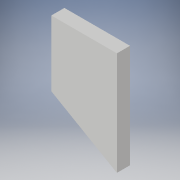
# Autodesk Inventor part: top right door
Saved by Autodesk Inventor 2017 (Build 210142000, 142)
## iProperties
Created: 2018-03-10
Part Number: top right door
Material: Generic
Document SubType Name: Modeling
Designer: Braxton
Density: 1 g/cm^3
Appearance: Default
Author: Braxton
Autodesk Inventor part; units mm, degrees
ref_plane "YZ Plane" through (0, 0, 0) normal (1, 0, 0) x (0, 1, 0)
ref_plane "XZ Plane" through (0, 0, 0) normal (0, 1, 0) x (-1, 0, 0)
ref_plane "XY Plane" through (0, 0, 0) normal (0, 0, 1) x (1, 0, 0)
sketch "Sketch1" plane through (0, 0, 0) normal (0, 0, 1) x (1, 0, 0)
  line L0 (1270, 1270) -> (1270, 2540)
  line L1 (1270, 1270) -> (2540, 536.7652)
  line L2 (2540, 536.7652) -> (2540, 2540)
  line L3 (2540, 2540) -> (1270, 2540)
  dimension "d448" = 2003.2348
  constraints: 8 end point
  measures "d448" distance of L1.end L2.end
extrude "door" add sketch "Sketch1" along normal mid plane 254
sketch "Sketch3" plane through (0, 0, 0) normal (0, 0, 1) x (1, 0, 0)
  line L0 (1295.4, 2436.0832) -> (1270, 2407.6852)
  line L1 (1295.4, 2461.4832) -> (1295.4, 2436.0832)
  line L2 (1270, 2448.7832) -> (1295.4, 2448.7832) construction
  line L3 (1270, 2489.8813) -> (1270, 2407.6852)
  line L4 (1270, 2489.8813) -> (1295.4, 2461.4832)
  line L5 (1295.4, 2271.691) -> (1270, 2243.2929)
  line L6 (1295.4, 2297.091) -> (1295.4, 2271.691)
  line L7 (1270, 2284.391) -> (1295.4, 2284.391) construction
  line L8 (1270, 2325.4891) -> (1270, 2243.2929)
  line L9 (1270, 2325.4891) -> (1295.4, 2297.091)
  line L10 (1244.6, 2353.8871) -> (1270, 2325.4891)
  line L11 (1270, 2366.5871) -> (1244.6, 2366.5871) construction
  line L12 (1244.6, 2379.2871) -> (1244.6, 2353.8871)
  line L13 (1244.6, 2379.2871) -> (1270, 2407.6852)
  line L14 (1270, 2407.6852) -> (1270, 2325.4891)
  line L15 (1295.4, 2107.2987) -> (1270, 2078.9007)
  line L16 (1295.4, 2132.6987) -> (1295.4, 2107.2987)
  line L17 (1270, 2119.9987) -> (1295.4, 2119.9987) construction
  line L18 (1270, 2161.0968) -> (1270, 2078.9007)
  line L19 (1270, 2161.0968) -> (1295.4, 2132.6987)
  line L20 (1244.6, 2189.4949) -> (1270, 2161.0968)
  line L21 (1270, 2202.1949) -> (1244.6, 2202.1949) construction
  line L22 (1244.6, 2214.8949) -> (1244.6, 2189.4949)
  line L23 (1244.6, 2214.8949) -> (1270, 2243.2929)
  line L24 (1270, 2243.2929) -> (1270, 2161.0968)
  line L25 (1295.4, 1942.9065) -> (1270, 1914.5084)
  line L26 (1295.4, 1968.3065) -> (1295.4, 1942.9065)
  line L27 (1270, 1955.6065) -> (1295.4, 1955.6065) construction
  line L28 (1270, 1996.7045) -> (1270, 1914.5084)
  line L29 (1270, 1996.7045) -> (1295.4, 1968.3065)
  line L30 (1244.6, 2025.1026) -> (1270, 1996.7045)
  line L31 (1270, 2037.8026) -> (1244.6, 2037.8026) construction
  line L32 (1244.6, 2050.5026) -> (1244.6, 2025.1026)
  line L33 (1244.6, 2050.5026) -> (1270, 2078.9007)
  line L34 (1270, 2078.9007) -> (1270, 1996.7045)
  line L35 (1295.4, 1778.5142) -> (1270, 1750.1162)
  line L36 (1295.4, 1803.9142) -> (1295.4, 1778.5142)
  line L37 (1270, 1791.2142) -> (1295.4, 1791.2142) construction
  line L38 (1270, 1832.3123) -> (1270, 1750.1162)
  line L39 (1270, 1832.3123) -> (1295.4, 1803.9142)
  line L40 (1244.6, 1860.7104) -> (1270, 1832.3123)
  line L41 (1270, 1873.4104) -> (1244.6, 1873.4104) construction
  line L42 (1244.6, 1886.1104) -> (1244.6, 1860.7104)
  line L43 (1244.6, 1886.1104) -> (1270, 1914.5084)
  line L44 (1270, 1914.5084) -> (1270, 1832.3123)
  line L45 (1295.4, 1614.122) -> (1270, 1585.7239)
  line L46 (1295.4, 1639.522) -> (1295.4, 1614.122)
  line L47 (1270, 1626.822) -> (1295.4, 1626.822) construction
  line L48 (1270, 1667.92) -> (1270, 1585.7239)
  line L49 (1270, 1667.92) -> (1295.4, 1639.522)
  line L50 (1244.6, 1696.3181) -> (1270, 1667.92)
  line L51 (1270, 1709.0181) -> (1244.6, 1709.0181) construction
  line L52 (1244.6, 1721.7181) -> (1244.6, 1696.3181)
  line L53 (1244.6, 1721.7181) -> (1270, 1750.1162)
  line L54 (1270, 1750.1162) -> (1270, 1667.92)
  line L55 (1295.4, 1449.7297) -> (1270, 1421.3317)
  line L56 (1295.4, 1475.1297) -> (1295.4, 1449.7297)
  line L57 (1270, 1462.4297) -> (1295.4, 1462.4297) construction
  line L58 (1270, 1503.5278) -> (1270, 1421.3317)
  line L59 (1270, 1503.5278) -> (1295.4, 1475.1297)
  line L60 (1244.6, 1531.9258) -> (1270, 1503.5278)
  line L61 (1270, 1544.6258) -> (1244.6, 1544.6258) construction
  line L62 (1244.6, 1557.3258) -> (1244.6, 1531.9258)
  line L63 (1244.6, 1557.3258) -> (1270, 1585.7239)
  line L64 (1270, 1585.7239) -> (1270, 1503.5278)
  line L65 (1244.6, 1392.9336) -> (1270, 1421.3317)
  line L66 (1270, 1380.2336) -> (1244.6, 1380.2336) construction
  line L67 (1244.6, 1392.9336) -> (1244.6, 1367.5336)
  line L68 (1270, 1421.3317) -> (1270, 1339.1355)
  line L69 (1244.6, 1367.5336) -> (1270, 1339.1355)
  line L70 (2540, 536.7652) -> (1270, 1270) projected
  line L71 (1531.5315, 1148.3341) -> (1543.4249, 1112.138)
  line L72 (1507.833, 1132.6871) -> (1520.533, 1154.6841) construction
  line L73 (1531.5315, 1148.3341) -> (1509.5344, 1161.0341)
  line L74 (1543.4249, 1112.138) -> (1472.241, 1153.2361)
  line L75 (1509.5344, 1161.0341) -> (1472.241, 1153.2361)
  line L76 (1472.241, 1153.2361) -> (1434.9475, 1145.4381)
  line L77 (1436.649, 1173.7851) -> (1423.949, 1151.7881) construction
  line L78 (1434.9475, 1145.4381) -> (1412.9505, 1158.1381)
  line L79 (1389.1636, 1230.5302) -> (1401.0571, 1194.3342)
  line L80 (1389.1636, 1230.5302) -> (1367.1666, 1243.2302)
  line L81 (1401.0571, 1194.3342) -> (1329.8731, 1235.4322)
  line L82 (1365.4651, 1214.8832) -> (1378.1651, 1236.8802) construction
  line L83 (1412.9505, 1158.1381) -> (1401.0571, 1194.3342)
  line L84 (1472.241, 1153.2361) -> (1401.0571, 1194.3342)
  line L85 (1367.1666, 1243.2302) -> (1329.8731, 1235.4322)
  line L86 (2267.1577, 664.9613) -> (2255.2643, 701.1574)
  line L87 (2289.1548, 652.2613) -> (2267.1577, 664.9613)
  line L88 (2290.8562, 680.6084) -> (2278.1562, 658.6113) construction
  line L89 (2326.4482, 660.0593) -> (2255.2643, 701.1574)
  line L90 (2326.4482, 660.0593) -> (2289.1548, 652.2613)
  line L91 (2243.3708, 737.3535) -> (2255.2643, 701.1574)
  line L92 (2219.6723, 721.7064) -> (2232.3723, 743.7035) construction
  line L93 (2243.3708, 737.3535) -> (2221.3738, 750.0535)
  line L94 (2255.2643, 701.1574) -> (2184.0803, 742.2555)
  line L95 (2221.3738, 750.0535) -> (2184.0803, 742.2555)
  line L96 (2184.0803, 742.2555) -> (2146.7869, 734.4575)
  line L97 (2148.4884, 762.8045) -> (2135.7884, 740.8075) construction
  line L98 (2146.7869, 734.4575) -> (2124.7898, 747.1575)
  line L99 (2124.7898, 747.1575) -> (2112.8964, 783.3535)
  line L100 (2184.0803, 742.2555) -> (2112.8964, 783.3535)
  line L101 (2101.003, 819.5496) -> (2112.8964, 783.3535)
  line L102 (2077.3044, 803.9026) -> (2090.0044, 825.8996) construction
  line L103 (2101.003, 819.5496) -> (2079.0059, 832.2496)
  line L104 (2112.8964, 783.3535) -> (2041.7125, 824.4516)
  line L105 (2041.7125, 824.4516) -> (2004.419, 816.6536)
  line L106 (2006.1205, 845.0006) -> (1993.4205, 823.0036) construction
  line L107 (2004.419, 816.6536) -> (1982.422, 829.3536)
  line L108 (1982.422, 829.3536) -> (1970.5285, 865.5497)
  line L109 (2041.7125, 824.4516) -> (1970.5285, 865.5497)
  line L110 (2079.0059, 832.2496) -> (2041.7125, 824.4516)
  line L111 (1958.6351, 901.7457) -> (1970.5285, 865.5497)
  line L112 (1934.9366, 886.0987) -> (1947.6366, 908.0957) construction
  line L113 (1958.6351, 901.7457) -> (1936.638, 914.4457)
  line L114 (1970.5285, 865.5497) -> (1899.3446, 906.6477)
  line L115 (1899.3446, 906.6477) -> (1862.0512, 898.8497)
  line L116 (1863.7526, 927.1968) -> (1851.0526, 905.1997) construction
  line L117 (1862.0512, 898.8497) -> (1840.0541, 911.5497)
  line L118 (1840.0541, 911.5497) -> (1828.1607, 947.7458)
  line L119 (1899.3446, 906.6477) -> (1828.1607, 947.7458)
  line L120 (1936.638, 914.4457) -> (1899.3446, 906.6477)
  line L121 (1816.2672, 983.9419) -> (1828.1607, 947.7458)
  line L122 (1792.5687, 968.2948) -> (1805.2687, 990.2919) construction
  line L123 (1816.2672, 983.9419) -> (1794.2702, 996.6419)
  line L124 (1828.1607, 947.7458) -> (1756.9767, 988.8439)
  line L125 (1794.2702, 996.6419) -> (1756.9767, 988.8439)
  line L126 (1756.9767, 988.8439) -> (1719.6833, 981.0458)
  line L127 (1721.3848, 1009.3929) -> (1708.6848, 987.3958) construction
  line L128 (1719.6833, 981.0458) -> (1697.6862, 993.7458)
  line L129 (1697.6862, 993.7458) -> (1685.7928, 1029.9419)
  line L130 (1756.9767, 988.8439) -> (1685.7928, 1029.9419)
  line L131 (1673.8994, 1066.138) -> (1685.7928, 1029.9419)
  line L132 (1650.2008, 1050.4909) -> (1662.9008, 1072.488) construction
  line L133 (1673.8994, 1066.138) -> (1651.9023, 1078.838)
  line L134 (1685.7928, 1029.9419) -> (1614.6089, 1071.04)
  line L135 (1651.9023, 1078.838) -> (1614.6089, 1071.04)
  line L136 (1579.0169, 1091.589) -> (1566.3169, 1069.592) construction
  line L137 (1577.3154, 1063.242) -> (1555.3184, 1075.942)
  line L138 (1555.3184, 1075.942) -> (1543.4249, 1112.138)
  line L139 (1614.6089, 1071.04) -> (1543.4249, 1112.138)
  line L140 (1614.6089, 1071.04) -> (1577.3154, 1063.242)
  line L141 (2409.5256, 582.7652) -> (2397.6321, 618.9613)
  line L142 (2431.5226, 570.0652) -> (2409.5256, 582.7652)
  line L143 (2433.2241, 598.4123) -> (2420.5241, 576.4152) construction
  line L144 (2468.8161, 577.8632) -> (2397.6321, 618.9613)
  line L145 (2468.8161, 577.8632) -> (2431.5226, 570.0652)
  line L146 (2385.7387, 655.1574) -> (2397.6321, 618.9613)
  line L147 (2362.0402, 639.5103) -> (2374.7402, 661.5074) construction
  line L148 (2363.7416, 667.8574) -> (2326.4482, 660.0593)
  line L149 (2385.7387, 655.1574) -> (2363.7416, 667.8574)
  line L150 (2397.6321, 618.9613) -> (2326.4482, 660.0593)
  line L151 (2528.1066, 572.9612) -> (2540, 536.7652)
  line L152 (2504.408, 557.3142) -> (2517.108, 579.3112) construction
  line L153 (2506.1095, 585.6612) -> (2468.8161, 577.8632)
  line L154 (2528.1066, 572.9612) -> (2506.1095, 585.6612)
  line L155 (2540, 536.7652) -> (2468.8161, 577.8632)
  constraints: 310 end point
extrude "connection give" add sketch "Sketch3" along normal mid plane 127 contours L68 L69 L67 L65 | L64 L60 L62 L63 | L54 L50 L52 L53 | L44 L40 L42 L43 | L34 L30 L32 L33 | L24 L20 L22 L23 | L14 L10 L12 L13 | L76 L78 L83 L70 | L140 L137 L138 L70 | L126 L128 L129 L70 | L115 L117 L118 L70 | L105 L107 L108 L70 | L96 L98 L99 L70 | L90 L87 L86 L70 | L145 L142 L141 L70
extrude "connection receive" cut sketch "Sketch3" along normal mid plane 127 contours L59 L56 L55 L58 | L49 L46 L45 L48 | L39 L36 L35 L38 | L29 L26 L25 L28 | L19 L16 L15 L18 | L9 L6 L5 L8 | L0 L3 L4 L1 | L70 L85 L80 L79 | L70 L75 L73 L71 | L70 L135 L133 L131 | L70 L125 L123 L121 | L70 L120 L113 L111 | L70 L110 L103 L101 | L70 L95 L93 L91 | L70 L148 L149 L146 | L70 L153 L154 L151
body "Solid1"
